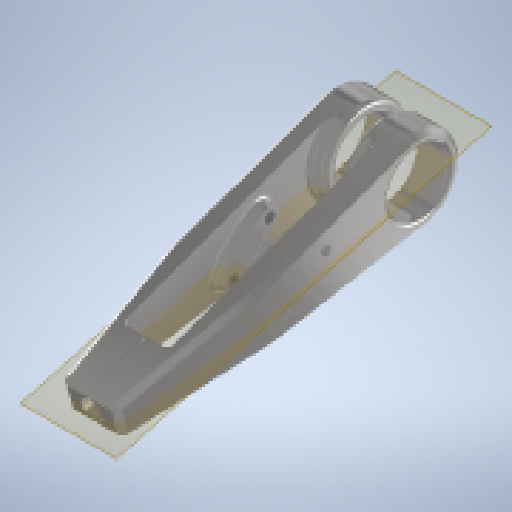
# Autodesk Inventor part: robotic_arm_part_3
Saved by Autodesk Inventor 2023 (Build 270158000, 158)
## iProperties
Created: 2023-11-19
Part Number: robotic_arm_part_3
Material: Steel, Mild
Document SubType Name: Modeling
Designer: Beatrice
Density: 7.85 g/cm^3
Appearance: Semi-Polished
Author: Beatrice
Autodesk Inventor part; units mm, degrees
ref_plane "YZ Plane" through (0, 0, 0) normal (1, 0, 0) x (0, 1, 0)
sketch "Sketch1" plane through (0, 0, 0) normal (1, 0, 0) x (0, 1, 0)
  line L0 (0, 109.23427) -> (0, -18.237146) construction
  line L1 (-54.087164, 0) -> (42.558374, 0)
  ellipse E0 centre (0.000415, 80.020843) end of major axis (0.000415, 77.016726) minor radius 3 (-0.022088, 77.016811) -> (0.022917, 77.016811) ccw
  line L2 (0.000631, 41.00085) -> (0, 41.00085) construction
  line L3 (2.467238, 42.251676) -> (-2.456164, 42.251676) construction
  ellipse E1 centre (0, 47.251435) end of major axis (4.2185, 47.251435) minor radius 4.212719 (4.2185, 47.251435) -> (-4.2185, 47.251435) ccw construction
  ellipse E2 centre (0, 47.251435) end of major axis (-3, 47.251435) minor radius 3 (0.022533, 44.251519) -> (-0.022533, 44.251519) ccw construction
  line L4 (0.000001, 91.024068) -> (0, 12.372435) construction
  ellipse E3 centre (0, 6.241435) end of major axis (-5, 6.241435) minor radius 5 construction
  ellipse E4 centre (0, 6.241435) end of major axis (6.25, 6.241435) minor radius 6.241435 (-6.242267, 6.551818) -> (6.239344, 6.605742) ccw construction
  line L5 (-4.20992, 47.251435) -> (-6.25, 6.241435) construction
  line L6 (4.221488, 47.251435) -> (6.244832, 6.495206) construction
  line L7 (-6.001619, 11.234435) -> (6.009553, 11.234435) construction
  line L8 (-2.456164, 42.251676) -> (-3.942535, 12.372435) construction
  line L9 (-3.942535, 12.372435) -> (3.950593, 12.372435) construction
  line L10 (-2.456674, 42.241435) -> (2.467746, 42.241435) construction
  line L11 (0.000627, 41.000095) -> (0, 41.000095) construction
  line L12 (2.467238, 42.251676) -> (3.950593, 12.372435) construction
  line L13 (-4.2185, 47.251435) -> (-4.20992, 47.251435) construction
  line L14 (0, 48.389405) -> (0, 48.389405) construction
  line L15 (3, 47.251435) -> (4.2185, 47.251435) construction
  line L16 (-19.109149, 33.389405) -> (19.109149, 33.389405) construction
  line L17 (-15.949888, 49.339293) -> (15.949888, 17.439516) construction
  line L18 (-15.99534, 17.394065) -> (15.99534, 49.384745) construction
  circle A0 centre (0, 47.251435) radius 3
  circle A1 centre (0, 47.251435) radius 4.2185
  line L19 (18.23022, 47.251435) -> (-40.280659, 47.251435) construction
  line L20 (-28.915137, 45.562681) -> (-28.915137, 48.940188) construction
  line L21 (0, 51.469935) -> (0, 43.032935) construction
  line L22 (0, 43.032935) -> (-28.915137, 45.562681) construction
  line L23 (0, 51.469935) -> (-28.915137, 48.940188) construction
  line L24 (-1.091828, 51.326193) -> (-28.366959, 41.398857)
  line L25 (-27.492796, 38.136436) -> (-28.366959, 41.398857)
  line L26 (1.091828, 43.176676) -> (-27.492796, 38.136436)
  line L27 (17.60904, 51.969763) -> (-38.908129, 36.826033) construction
  line L28 (-1.091828, 51.326193) -> (1.091828, 43.176676) construction
  line L29 (-11.845739, 45.235144) -> (-12.729622, 44.35126)
  line L30 (-12.729622, 44.35126) -> (-10.961855, 42.583493)
  line L31 (-10.961855, 42.583493) -> (-10.077972, 43.467377)
  line L32 (-11.845739, 45.235144) -> (-10.961855, 46.119027)
  line L33 (-10.961855, 46.119027) -> (-9.194088, 44.35126)
  line L34 (-9.194088, 44.35126) -> (-10.077972, 43.467377)
  line L35 (-34.002813, 47.251435) -> (-25.278291, 38.526913)
  line L36 (-21.561378, 39.182305) -> (-22.707266, 43.458817)
  line L37 (-28.188696, 40.733572) -> (-22.393141, 42.286487)
  line L38 (-27.671058, 38.801721) -> (-21.875503, 40.354635)
  line L39 (-13.402845, 41.866428) -> (-9.161157, 46.108116) construction
  circle A2 centre (-9.161157, 46.108116) radius 0.5
  circle A3 centre (-9.161157, 46.108116) radius 0.9
  line L40 (-10.961855, 46.119027) -> (-9.606243, 46.890355)
  line L41 (-9.194088, 44.35126) -> (-8.396947, 45.63274)
  circle A4 centre (-12.718711, 42.550562) radius 0.5
  circle A5 centre (-12.718711, 42.550562) radius 0.9
  line L42 (-12.729622, 44.35126) -> (-13.50095, 42.995648)
  line L43 (-10.961855, 42.583493) -> (-12.243335, 41.786351)
  point P0 (28.751869, 36.37116)
  point P1 (0, 0)
  point P2 (-6.009, 41)
  point P3 (0, 33.389405)
  point P4 (0, 47.251435)
  point P5 (0, 47.251435)
  point P6 (-1.091834, 51.326191)
  point P7 (0.367667, 43.048987)
  point P8 (-1.78281, 51.074696)
  point P9 (-23.281172, 39.977987)
  dimension "d33" = 3
  dimension "d34" = 5
  dimension "d35" = 6.24143
  dimension "d13" = 41.01
  dimension "d15" = 6.24143
  dimension "d20" = 4.993
  dimension "d21" = 5.69
  dimension "d23" = 29.869
  dimension "d24" = 1.138
  dimension "d27" = 2
  dimension "d32" = 90
  dimension "d44" = 15
  dimension "d46" = 2.5
  dimension "d47" = 1.25
  dimension "d48" = 60
  dimension "d49" = 2
  dimension "d50" = 1
  dimension "d57" = 6
  dimension "d65" = 1
  dimension "d66" = 1.8
  constraints: 84 end point, 25 point on line, 8 coincident, 7 parallel, 7 symmetric about line, 5 centre point, 4 midpoint, 4 perpendicular, 4 point on circle, 3 horizontal, 2 horizontal alignment, 2 tangent, 45 other
  measures "d13" distance of point (0, 47.251) point (0, 6.241)
  measures "d15" distance of point (0, 0) point (0, 6.241)
  measures "d20" distance from line of point (0, 6.241) L7
  measures "d21" angle of L5 L6
  measures "d23" distance between parallel lines of L9 L10
  measures "d24" distance between parallel lines of L7 L9
  measures "d27" distance between parallel lines of L5 L8
  measures "d32" angle of L17 L18
  measures "d46" distance between parallel lines of L29 L31
  measures "d47" distance between parallel lines of L17 L30
  measures "d48" angle of L35 L27
  measures "d49" distance between parallel lines of L38 L37
  measures "d50" distance between parallel lines of L37 L27
  measures "d57" distance between parallel lines of L36 L25
  measures "d65" diameter of A2
  measures "d66" diameter of A3
extrude "Extrusion1" add sketch "Sketch1" against normal blind 2 contours A1 L26 L24 | A1 L26 L36 L24 | L36 L37 L35 L24 | L26 L35 L38 L36 | L35 L37 L25 L24 | L36 L38 L35 L37 | L26 L25 L38 L35 | L35 L38 L25 L37 | L32 L33 L34 L31 L30 L29 | L30 L43 A5 L42 | L40 A3 L41 L33 | A5 | A3 | A2 | A4
extrude "Extrusion2" add sketch "Sketch1" along normal blind 1.5 contours A1 L26 L24
extrude "Extrusion3" add sketch "Sketch1" along normal blind 2.3 contours L36 L37 L35 L24 | L26 L35 L38 L36 | L35 L37 L25 L24 | L36 L38 L35 L37 | L26 L25 L38 L35 | L35 L38 L25 L37
ref_plane "Work Plane1" through (2.3, 0, 0) normal (1, 0, 0) x (0, 0, -1)
extrude "Extrusion4" add sketch "Sketch1" along normal blind 2.3 contours L32 L33 L34 L31 L30 L29
sketch "Sketch2" plane through (2.3, -9.194088, 44.35126) normal (0, 0.7071068, -0.7071068) x (-1, 0, 0)
  line L0 (4.3, -5.130737) -> (2.3, -5.130737)
  line L1 (2.3, -5.130737) -> (2.3, -2.5)
  line L2 (2.3, -2.5) -> (0, -2.5)
  line L3 (0, -2.5) -> (0, 0)
  line L4 (0, 0) -> (2.3, 0)
  line L5 (2.3, 0) -> (2.3, 8.951712)
  line L6 (2.3, 8.951712) -> (4.3, 8.951712)
  line L7 (4.3, 8.951712) -> (4.3, -5.130737)
  line L8 (2.3, -2.5) -> (2.3, 0)
  line L9 (0, 0) -> (0, -2.5)
  line L10 (0, -1.25) -> (2.3, -1.25) construction
  line L11 (2.3, 0) -> (0, 0)
  line L12 (1.15, 0) -> (1.15, -2.5) construction
  line L13 (2.3, -2.5) -> (0, -2.5)
  circle A0 centre (0, -1.25) radius 0.9
  point P0 (2.3, -24.859875)
  point P1 (0, -0.35)
  point P2 (0, -2.15)
  dimension "d62" = 1.8
  constraints: 4 end point, 4 midpoint, 1 centre point, 1 coincident
  measures "d62" diameter of A0
extrude "Extrusion5" cut sketch "Sketch2" against normal blind 1.5 contours L3 A0 picked at (0.234549, -1.062953)
hole "Hole1" at (0, 28.751869, 36.37116) at (0, 6.239344, 6.605742) at (0, -9.161157, 46.108116) at (0, -12.718711, 42.550562) direction (-1, 0, 0) diameter 1 end through all
extrude "Extrusion6" add sketch "Sketch1" along normal blind 1 contours L30 L43 A5 L42 | L40 A3 L41 L33 | A5 | A3
thread "Thread1" size "M1x0.25" class "6H" standard "ANSI Metric M Profile" full length
thread "Thread2" size "M1x0.25" class "6H" standard "ANSI Metric M Profile" full length
sketch "Sketch3" plane through (0, -22.707266, 43.458817) normal (0, 0.9659258, 0.258819) x (1, 0, 0)
  line L0 (2.3, 4.427371) -> (2.3, 0)
  line L1 (2.3, 0) -> (0, 0)
  line L2 (0, 4.427371) -> (0, 0)
  line L3 (-2, 4.427371) -> (0, 4.427371)
  line L4 (-2, 0) -> (-2, 4.427371)
  line L5 (0, 0) -> (-2, 0)
  line L6 (0, 4.427371) -> (2.3, 4.427371)
  line L7 (2.3, 0.524932) -> (2.3, 3.902439)
  line L8 (2.3, 2.213685) -> (-2, 2.213685)
  line L9 (-2, 3.902439) -> (-2, 0.524932)
  circle A0 centre (2.3, 2.213685) radius 1.020674
  circle A1 centre (2.3, 2.213685) radius 0.5
  point P0 (0, 47.855066)
  point P1 (2.3, 1.713685)
  point P2 (2.3, 2.713685)
  dimension "d83" = 1
  constraints: 2 centre point, 2 coincident, 2 end point, 2 midpoint
  measures "d83" diameter of A1
ref_plane "Work Plane2" through (0, -26.57097, 42.423541) normal (0, 0.9659258, 0.258819) x (1, 0, 0)
sketch "Sketch4" plane through (0, -26.57097, 42.423541) normal (0, 0.9659258, 0.258819) x (1, 0, 0)
  line L0 (2.3, 4.077416) -> (2.3, 0.349955)
  line L1 (2.3, 0.349955) -> (-2, 0.349955)
  line L2 (-2, 0.349955) -> (-2, 4.077416)
  line L3 (-2, 4.077416) -> (2.3, 4.077416)
  circle A0 centre (2.3, 2.213685) radius 1.020674
  point P0 (0, 47.855066)
  point P1 (2.3, 1.193011)
  point P2 (2.3, 3.23436)
extrude "Extrusion7" cut sketch "Sketch4" against normal through all contours L0 A0 picked at (2.020001, 2.020415)
extrude "Extrusion8" cut sketch "Sketch3" against normal blind 10 contours L0 L8 A1 | L0 A1 L8
thread "Thread3" size "M1x0.25" class "6H" standard "ANSI Metric M Profile" full length
mirror "Mirror1" about plane through (2.3, 0, 0) normal (1, 0, 0) of "Extrusion1", "Extrusion2", "Extrusion3", "Extrusion4", "Extrusion5", "Hole1", "Extrusion6", "Extrusion7", "Extrusion8"
sketch "Sketch5" plane through (-2, -1.091834, 51.326191) normal (0, -0.3420202, 0.9396926) x (1, 0, 0)
  line L0 (0, 0) -> (3.5, 0)
  line L1 (0, -29.025582) -> (0, 0)
  line L2 (0, -29.025582) -> (8.6, -29.025582)
  line L3 (8.6, -29.025582) -> (8.6, 0)
  line L4 (8.6, 0) -> (5.1, 0)
  line L5 (5.1, 0) -> (5.1, -0.735322)
  line L6 (6.6, -0.735322) -> (5.1, -0.735322)
  line L7 (6.6, -0.735322) -> (6.6, -23.002663)
  line L8 (2, -23.002663) -> (6.6, -23.002663)
  line L9 (2, -0.735322) -> (2, -23.002663)
  line L10 (2, -0.735322) -> (3.5, -0.735322)
  line L11 (3.5, 0) -> (3.5, -0.735322)
  line L12 (0, -29.319951) -> (8.6, -29.319951)
  line L13 (4.3, -29.025582) -> (4.3, -23.002663)
  line L14 (6.963841, -29.319951) -> (8.6, -16)
  line L15 (7, -29.025582) -> (8.6, -29.025582)
  line L16 (8.6, -15.841023) -> (8.6, -29.319951)
  line L17 (0, -29.319951) -> (0, 0)
  line L18 (1.636159, -29.319951) -> (0, -16)
  line L19 (1.6, -29.025582) -> (0, -29.025582)
  line L20 (8.6, -29.319951) -> (0, -29.319951)
  point P0 (2, -16.528604)
  point P1 (0, -16)
  constraints: 16 end point, 11 point on line, 3 symmetric about line, 2 midpoint, 1 horizontal, 1 perpendicular
extrude "Extrusion9" cut sketch "Sketch5" against normal blind 10 contours L18 L2 L1 | L2 L18 L12 L17 | L14 L3 L2 | L2 L16 L12 L14
chamfer "Chamfer1" distance 0.5 angle 45 6 edges at (6.6, -8.6094, 48.59) (6.6, -6.5405, 41.8309) (6.6, 4.0748, 48.3433) (-2, -8.6094, 48.59) (-2, 4.0748, 48.3433) (-2, -6.5405, 41.8309)
chamfer "Chamfer2" distance 0.5 angle 45 8 edges at (5.55, -24.1594, 42.9303) (5.5319, -22.8681, 38.9519) (4.9819, -27.9299, 39.7676) (2.3, -28.367, 41.3989) (2.3, -27.4928, 38.1364) (-0.3819, -27.9299, 39.7676) (-0.95, -24.1594, 42.9303) (-0.9319, -22.8681, 38.9519)
fillet "Fillet1" radius 0.5 12 edges at (0, -22.1343, 41.3206) (4.6, -22.1343, 41.3206) (0, -4.0748, 46.1596) (4.6, -4.0748, 46.1596) (3.1, -4.0748, 46.1596) (3.1, 4.0748, 48.3433) (3.1, -1.4373, 51.2004) (1.5, 4.0748, 48.3433) (1.5, -4.0748, 46.1596) (1.5, -1.4373, 51.2004) (1.5, 0.7297, 43.1128) (3.1, 0.7297, 43.1128)
fillet "Fillet2" radius 0.5 4 edges at (-2, -3, 47.2514) (1.5, -3, 47.2514) (6.6, -3, 47.2514) (3.1, -3, 47.2514)
fillet "Fillet3" radius 0.5 16 edges at (0, -13.3425, 41.9018) (0, -13.1153, 43.6735) (0, -11.6026, 42.1849) (0, -10.078, 43.4674) (0, -8.5124, 46.7319) (0, -10.284, 46.5047) (0, -8.7955, 44.992) (0, -11.8457, 45.2351) (4.6, -10.284, 46.5047) (4.6, -8.7955, 44.992) (4.6, -8.5124, 46.7319) (4.6, -11.8457, 45.2351) (4.6, -13.3425, 41.9018) (4.6, -11.6026, 42.1849) (4.6, -13.1153, 43.6735) (4.6, -10.078, 43.4674)
sketch "Sketch6" plane through (0.105382, -28.237549, 40.915894) normal (0, -0.9659258, -0.258819) x (1, 0, 0)
  circle A0 centre (2.194618, -1.188753) radius 1.020674
  line L0 (4.389237, 0) -> (4.363784, -2.377507)
  line L1 (0, 0) -> (4.389237, 0)
  line L2 (0.025453, -2.377507) -> (0, 0)
  line L3 (4.363784, -2.377507) -> (0.025453, -2.377507)
  line L4 (2.144618, -8.377507) -> (2.244618, -8.377507)
  line L5 (2.244618, -8.377507) -> (2.244618, 6)
  line L6 (2.244618, 6) -> (2.144618, 6)
  line L7 (2.144618, 6) -> (2.144618, -8.377507)
  line L8 (2.144618, -8.377507) -> (2.244618, 6) construction
  line L9 (2.244618, -8.377507) -> (2.144618, 6) construction
  point P0 (-0.105382, -46.830134)
  dimension "d99" = 0.1
  constraints: 12 end point, 2 midpoint, 2 parallel, 1 horizontal, 1 perpendicular
  measures "d99" distance of L6.end L5.end
extrude "Extrusion10" cut sketch "Sketch6" against normal through all contours L5 A0 L7 | A0 L7 L1 L5 | L5 L3 L7 A0 | L1 L7 L6 L5 | L5 L4 L7 L3
chamfer "Chamfer3" distance 0.1 angle 45 19 edges at (2.25, -25.3022, 42.5143) (2.35, -25.3022, 42.5143) (2.35, -27.3113, 38.4213) (2.25, -27.3113, 38.4213) (2.25, -11.8457, 45.2351) (2.35, -11.8457, 45.2351) (2.25, -11.8457, 43.4674) (2.35, -11.8457, 43.4674) (2.25, -10.078, 45.2351) (2.35, -10.078, 45.2351) (2.35, -24.2809, 38.7028) (2.25, -21.7835, 40.0112) (2.35, -21.7835, 40.0112) (2.35, -22.4852, 42.63) (2.25, -22.4852, 42.63) (2.25, -24.2809, 38.7028) (2.35, -28.2156, 40.8341) (2.25, -28.0673, 41.2429) (2.35, -28.0673, 41.2429)
ref_plane "Work Plane3" through (-1.5, -46.574697, 34.771782) normal (0, -0.2588191, 0.9659258) x (-1, 0, 0)
ref_plane "Work Plane4" through (2.3, -14.346493, 40.962197) normal (1, 0, 0) x (0, 0.1736482, -0.9848078)
sketch "Sketch7" plane through (1, 1.091828, 43.176676) normal (0, 0.1736482, -0.9848078) x (-1, 0, 0)
  point P0 (1, -8.572792)
body "Solid1"
